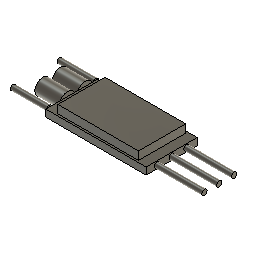
Battle bot V3,6 (Autodesk Fusion 360 archive; units mm, degrees)
design "40a esc brushless"
Autodesk Fusion 360 part; units mm, degrees
sketch "Sketch1" plane through (0, 0, 0) normal (0, 0, 1) x (1, 0, 0)
  line L0 (0, 0) -> (52.74, 0)
  line L1 (52.74, 0) -> (52.74, 26.87)
  line L2 (52.74, 26.87) -> (0, 26.87)
  line L3 (0, 26.87) -> (0, 0)
  dimension "d1" = 52.74
  dimension "d2" = 26.87
  constraint horizontal L0
  constraint vertical L1
  constraint horizontal L2
  constraint vertical L3
  constraint coincident L0.start L3.end
  measures "d1" distance of L0.start L0.end
  measures "d2" distance of L0 L2
extrude "Extrude1" add sketch "Sketch1" along normal blind 3.7
sketch "Sketch2" plane through (0, 0, 0) normal (-1, 0, 0) x (0, -1, 0)
  line L0 (-26.87, 0) -> (0, 0)
  line L1 (0, 0) -> (0, 3.7)
  line L2 (0, 3.7) -> (-26.87, 3.7)
  line L3 (-26.87, 3.7) -> (-26.87, 0)
  circle A0 centre (-20.65, 1.85) radius 4.12
  line L4 (-20.65, 1.85) -> (-11.35, 1.85) construction
  circle A1 centre (-11.35, 1.85) radius 4.12
  circle A2 centre (-26.2658, 3.1834) radius 1.4
  circle A3 centre (-1.7767, 3.1834) radius 1.4
  dimension "d5" = 8.24
  dimension "d6" = 6.22
  dimension "d7" = 9.3
  dimension "d8" = 8.24
  dimension "d9" = 2.8
  dimension "d10" = 2.8
  constraint coincident A0.centre L4.start
  constraint perpendicular L1 L4
  constraint coincident L4.end A1.centre
  measures "d5" diameter of A0
  measures "d6" distance of L3 A0.centre
  measures "d7" distance of A0.centre L4.end
  measures "d8" diameter of A1
  measures "d9" diameter of A2
  measures "d10" diameter of A3
extrude "Extrude2" add sketch "Sketch2" along normal blind 13 contours L0 L2 A0 | L0 A0 | L2 L3 A2 | L2 L3 A2 | L2 A0 | L0 L2 A1 | L0 A1 | L2 A1 | L2 A3 | L2 A3
extrude "Extrude3" add 2 faces at (-13, 26.6777, 2.866) (-13, 1.2269, 3.5008) along direction (-1, 0, 0) blind 6
sketch "Sketch3" plane through (0, 0, 3.7) normal (0, 0, 1) x (-1, 0, 0)
  line L0 (0, -26.87) -> (0, -24.9646)
  line L1 (0, -24.9646) -> (0, -24.3313)
  line L2 (0, -24.3313) -> (0, -16.9687)
  line L3 (0, -16.9687) -> (0, -15.0313)
  line L4 (0, -15.0313) -> (0, -7.6687)
  line L5 (0, -7.6687) -> (0, -3.0779)
  line L6 (0, -3.0779) -> (0, -0.4755)
  line L7 (0, -0.4755) -> (0, 0)
  line L8 (0, 0) -> (-52.74, 0)
  line L9 (-52.74, 0) -> (-52.74, -26.87)
  line L10 (-52.74, -26.87) -> (0, -26.87)
  line L11 (-47.74, -1) -> (-5.34, -1)
  line L12 (-5.34, -1) -> (-5.34, -25.76)
  line L13 (-5.34, -25.76) -> (-47.74, -25.76)
  line L14 (-47.74, -25.76) -> (-47.74, -1)
  dimension "d15" = 24.76
  dimension "d16" = 1
  dimension "d17" = 42.4
  dimension "d18" = 5
  constraint horizontal L11
  constraint vertical L12
  constraint horizontal L13
  constraint vertical L14
  measures "d15" distance of L11 L13
  measures "d16" distance of L8 L11
  measures "d17" distance of L12 L14
  measures "d18" distance of L9 L14
extrude "Extrude4" add sketch "Sketch3" along normal blind 4.3 contours L11 L12 L13 L14
sketch "Sketch4" plane through (52.74, 0, 0) normal (1, 0, 0) x (0, 1, 0)
  line L0 (0, 0) -> (26.87, 0)
  line L1 (26.87, 0) -> (26.87, 3.7)
  line L2 (26.87, 3.7) -> (0, 3.7)
  line L3 (0, 3.7) -> (0, 0)
  circle A0 centre (13.435, 1.85) radius 1.4
  line L4 (14.835, 1.85) -> (19.835, 1.85) construction
  circle A1 centre (21.235, 1.85) radius 1.4
  line L5 (13.435, 1.85) -> (13.435, 3.7) construction
  circle A2 centre (5.635, 1.85) radius 1.4
  dimension "d21" = 2.8
  dimension "d22" = 5
  dimension "d23" = 2.8
  constraint coincident A0 L4.start
  constraint parallel L2 L4
  constraint coincident L4.end A1
  constraint coincident A0.centre L5.start
  constraint midpoint L2 L5.end
  constraint perpendicular L2 L5
  constraint symmetric A1 L5 A2
  measures "d21" diameter of A0
  measures "d22" distance of L4.start L4.end
  measures "d23" diameter of A1
extrude "Extrude5" add sketch "Sketch4" along normal blind 25 contours A0 | A1 | A2

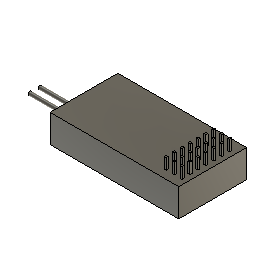
design "Reciever"
Autodesk Fusion 360 part; units mm, degrees
sketch "Sketch1" plane through (0, 0, 0) normal (0, 0, 1) x (1, 0, 0)
  line L0 (0, 0) -> (41.17, 0)
  line L1 (41.17, 0) -> (41.17, 21.69)
  line L2 (41.17, 21.69) -> (0, 21.69)
  line L3 (0, 21.69) -> (0, 0)
  dimension "d1" = 41.17
  dimension "d2" = 21.69
  constraint horizontal L0
  constraint vertical L1
  constraint horizontal L2
  constraint vertical L3
  constraint coincident L0.start L3.end
  measures "d1" distance of L0.start L0.end
  measures "d2" distance of L0.start L2.end
extrude "Extrude1" add sketch "Sketch1" along normal blind 8.92
sketch "Sketch2" plane through (0, 0, 8.92) normal (0, 0, 1) x (-1, 0, 0)
  line L0 (0, -21.69) -> (0, 0)
  line L1 (0, 0) -> (-41.17, 0)
  line L2 (-41.17, 0) -> (-41.17, -21.69)
  line L3 (-41.17, -21.69) -> (0, -21.69)
  line L4 (-33.97, -18.44) -> (-39.67, -18.44)
  line L5 (-39.67, -18.44) -> (-39.67, -2.54)
  line L6 (-39.67, -2.54) -> (-33.97, -2.54)
  line L7 (-33.97, -2.54) -> (-33.97, -18.44)
  line L8 (-39.67, -18.44) -> (-39.02, -18.44)
  line L9 (-39.02, -18.44) -> (-39.02, -17.79)
  line L10 (-39.02, -17.79) -> (-39.67, -17.79)
  line L11 (-39.67, -17.79) -> (-39.67, -18.44)
  line L12 (-37.145, -18.44) -> (-36.495, -18.44)
  line L13 (-36.495, -18.44) -> (-36.495, -17.79)
  line L14 (-37.145, -17.79) -> (-37.145, -18.44)
  line L15 (-36.495, -17.79) -> (-37.145, -17.79)
  line L16 (-34.62, -18.44) -> (-33.97, -18.44)
  line L17 (-33.97, -18.44) -> (-33.97, -17.79)
  line L18 (-34.62, -17.79) -> (-34.62, -18.44)
  line L19 (-33.97, -17.79) -> (-34.62, -17.79)
  line L20 (-39.67, -15.8983) -> (-39.02, -15.8983)
  line L21 (-39.02, -15.8983) -> (-39.02, -15.2483)
  line L22 (-39.67, -15.2483) -> (-39.67, -15.8983)
  line L23 (-39.02, -15.2483) -> (-39.67, -15.2483)
  line L24 (-37.145, -15.8983) -> (-36.495, -15.8983)
  line L25 (-36.495, -15.8983) -> (-36.495, -15.2483)
  line L26 (-37.145, -15.2483) -> (-37.145, -15.8983)
  line L27 (-36.495, -15.2483) -> (-37.145, -15.2483)
  line L28 (-34.62, -15.8983) -> (-33.97, -15.8983)
  line L29 (-33.97, -15.8983) -> (-33.97, -15.2483)
  line L30 (-34.62, -15.2483) -> (-34.62, -15.8983)
  line L31 (-33.97, -15.2483) -> (-34.62, -15.2483)
  line L32 (-39.67, -13.3567) -> (-39.02, -13.3567)
  line L33 (-39.02, -13.3567) -> (-39.02, -12.7067)
  line L34 (-39.67, -12.7067) -> (-39.67, -13.3567)
  line L35 (-39.02, -12.7067) -> (-39.67, -12.7067)
  line L36 (-37.145, -13.3567) -> (-36.495, -13.3567)
  line L37 (-36.495, -13.3567) -> (-36.495, -12.7067)
  line L38 (-37.145, -12.7067) -> (-37.145, -13.3567)
  line L39 (-36.495, -12.7067) -> (-37.145, -12.7067)
  line L40 (-34.62, -13.3567) -> (-33.97, -13.3567)
  line L41 (-33.97, -13.3567) -> (-33.97, -12.7067)
  line L42 (-34.62, -12.7067) -> (-34.62, -13.3567)
  line L43 (-33.97, -12.7067) -> (-34.62, -12.7067)
  line L44 (-39.67, -10.815) -> (-39.02, -10.815)
  line L45 (-39.02, -10.815) -> (-39.02, -10.165)
  line L46 (-39.67, -10.165) -> (-39.67, -10.815)
  line L47 (-39.02, -10.165) -> (-39.67, -10.165)
  line L48 (-37.145, -10.815) -> (-36.495, -10.815)
  line L49 (-36.495, -10.815) -> (-36.495, -10.165)
  line L50 (-37.145, -10.165) -> (-37.145, -10.815)
  line L51 (-36.495, -10.165) -> (-37.145, -10.165)
  line L52 (-34.62, -10.815) -> (-33.97, -10.815)
  line L53 (-33.97, -10.815) -> (-33.97, -10.165)
  line L54 (-34.62, -10.165) -> (-34.62, -10.815)
  line L55 (-33.97, -10.165) -> (-34.62, -10.165)
  line L56 (-39.67, -8.2733) -> (-39.02, -8.2733)
  line L57 (-39.02, -8.2733) -> (-39.02, -7.6233)
  line L58 (-39.67, -7.6233) -> (-39.67, -8.2733)
  line L59 (-39.02, -7.6233) -> (-39.67, -7.6233)
  line L60 (-37.145, -8.2733) -> (-36.495, -8.2733)
  line L61 (-36.495, -8.2733) -> (-36.495, -7.6233)
  line L62 (-37.145, -7.6233) -> (-37.145, -8.2733)
  line L63 (-36.495, -7.6233) -> (-37.145, -7.6233)
  line L64 (-34.62, -8.2733) -> (-33.97, -8.2733)
  line L65 (-33.97, -8.2733) -> (-33.97, -7.6233)
  line L66 (-34.62, -7.6233) -> (-34.62, -8.2733)
  line L67 (-33.97, -7.6233) -> (-34.62, -7.6233)
  line L68 (-39.67, -5.7317) -> (-39.02, -5.7317)
  line L69 (-39.02, -5.7317) -> (-39.02, -5.0817)
  line L70 (-39.67, -5.0817) -> (-39.67, -5.7317)
  line L71 (-39.02, -5.0817) -> (-39.67, -5.0817)
  line L72 (-37.145, -5.7317) -> (-36.495, -5.7317)
  line L73 (-36.495, -5.7317) -> (-36.495, -5.0817)
  line L74 (-37.145, -5.0817) -> (-37.145, -5.7317)
  line L75 (-36.495, -5.0817) -> (-37.145, -5.0817)
  line L76 (-34.62, -5.7317) -> (-33.97, -5.7317)
  line L77 (-33.97, -5.7317) -> (-33.97, -5.0817)
  line L78 (-34.62, -5.0817) -> (-34.62, -5.7317)
  line L79 (-33.97, -5.0817) -> (-34.62, -5.0817)
  line L80 (-39.67, -3.19) -> (-39.02, -3.19)
  line L81 (-39.02, -3.19) -> (-39.02, -2.54)
  line L82 (-39.67, -2.54) -> (-39.67, -3.19)
  line L83 (-39.02, -2.54) -> (-39.67, -2.54)
  line L84 (-37.145, -3.19) -> (-36.495, -3.19)
  line L85 (-36.495, -3.19) -> (-36.495, -2.54)
  line L86 (-37.145, -2.54) -> (-37.145, -3.19)
  line L87 (-36.495, -2.54) -> (-37.145, -2.54)
  line L88 (-34.62, -3.19) -> (-33.97, -3.19)
  line L89 (-33.97, -3.19) -> (-33.97, -2.54)
  line L90 (-34.62, -2.54) -> (-34.62, -3.19)
  line L91 (-33.97, -2.54) -> (-34.62, -2.54)
  dimension "d5" = 5.7
  dimension "d6" = 15.9
  dimension "d7" = 1.5
  dimension "d8" = 3.25
  dimension "d9" = 0.65
  dimension "d10" = 0.65
  dimension "d13" = 5.05
  dimension "d14" = 15.25
  constraint horizontal L4
  constraint vertical L5
  constraint horizontal L6
  constraint vertical L7
  constraint horizontal L8
  constraint vertical L9
  constraint horizontal L10
  constraint vertical L11
  measures "d5" distance of L4.start L4.end
  measures "d6" distance of L4.start L6.end
  measures "d7" distance of L2 L5
  measures "d8" distance of L3 L4
  measures "d9" distance of L4.end L8.end
  measures "d10" distance of L4.end L10.end
extrude "Extrude2" add sketch "Sketch2" along normal blind 3.5 contours L4 L7 L16 L17 L18 L19 | L4 L12 L13 L14 L15 | L7 L28 L29 L30 L31 | L4 L5 L8 L9 L10 L11 | L7 L40 L41 L42 L43 | L7 L52 L53 L54 L55 | L5 L20 L21 L22 L23 | L7 L64 L65 L66 L67 | L5 L32 L33 L34 L35 | L7 L76 L77 L78 L79 | L5 L44 L45 L46 L47 | L6 L7 L88 L89 L90 L91 | L5 L56 L57 L58 L59 | L5 L68 L69 L70 L71 | L6 L84 L85 L86 L87 | L5 L6 L80 L81 L82 L83 | L24 L25 L26 L27 | L36 L37 L38 L39 | L48 L49 L50 L51 | L60 L61 L62 L63 | L72 L73 L74 L75
sketch "Sketch3" plane through (0, 0, 0) normal (-1, 0, 0) x (0, -1, 0)
  line L0 (-21.69, 0) -> (0, 0)
  line L1 (0, 0) -> (0, 8.92)
  line L2 (0, 8.92) -> (-21.69, 8.92)
  line L3 (-21.69, 8.92) -> (-21.69, 0)
  circle A0 centre (-9.85, 4.4059) radius 0.6
  circle A1 centre (-6.57, 4.4059) radius 0.6
  line L4 (-5.97, 4.4059) -> (-10.45, 4.4059) construction
  dimension "d17" = 1.2
  dimension "d18" = 11.84
  dimension "d19" = 1.2
  dimension "d20" = 4.48
  constraint coincident A1 L4.start
  constraint coincident A0 L4.end
  constraint horizontal L4
  measures "d17" diameter of A0
  measures "d18" distance of L3 A0.centre
  measures "d19" diameter of A1
  measures "d20" distance of L4.start L4.end
extrude "Extrude3" add sketch "Sketch3" along normal blind 13 contours A0 | A1

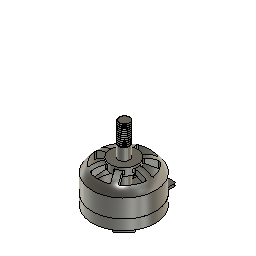
design "Weapon motor"
Autodesk Fusion 360 part; units mm, degrees
sketch "Sketch1" plane through (0, 0, 0) normal (0, 0, 1) x (1, 0, 0)
  circle A0 centre (0, 0) radius 2.5
  dimension "d1" = 5
  constraint coincident A0.centre origin
  measures "d1" diameter of A0
extrude "Extrude1" add sketch "Sketch1" along normal blind 33.45 makes body 1
ref_plane "WorkPlane1" through (0, 0, 19.34) normal (0, 0, 1) x (1, 0, 0)
sketch "Sketch2" plane through (0, 0, 19.34) normal (0, 0, 1) x (1, 0, 0)
  circle A0 centre (0, 0) radius 5.935
  dimension "d5" = 11.87
  constraint coincident A0.centre origin
  measures "d5" diameter of A0
extrude "Extrude2" add sketch "Sketch2" against normal blind 0.98 bodies 1
sketch "Sketch3" plane through (0, 0, 18.36) normal (0, 0, -1) x (1, 0, 0)
  circle A0 centre (0, 0) radius 5.935
  circle A1 centre (0, 0) radius 2.5
  circle A2 centre (0, 0) radius 13.905
  dimension "d8" = 27.81
  constraint concentric A0 A2
  measures "d8" diameter of A2
ref_plane "WorkPlane2" through (0, 0, 45.735) normal (0, 1, 0) x (0, 0, 1)
sketch "Sketch4" plane through (0, 0, 45.735) normal (0, 1, 0) x (1, 0, 0)
  line L0 (-2.5, 26.395) -> (2.5, 26.395)
  line L1 (-2.5, 12.285) -> (2.5, 12.285)
  line L2 (5.935, 27.375) -> (-5.935, 27.375)
  line L3 (-5.935, 26.395) -> (5.935, 26.395)
  line L4 (-2.5, 45.735) -> (2.5, 45.735)
  line L5 (2.5, 27.375) -> (-2.5, 27.375)
  line L6 (2.5, 27.375) -> (2.5, 32.315) construction
  line L7 (0, 27.375) -> (13.9, 27.375) construction
  line L8 (-2.5, 26.395) -> (-2.5, 45.645) construction
  line L9 (-2.5, 45.735) -> (-2.5, 43.865) construction
  line L10 (13.9, 32.315) -> (13.9, 40.315)
  arc A0 (5.935, 27.375) -> (13.9, 32.315) centre (5.935, 36.2662) ccw
  line L11 (11.4, 32.315) -> (11.4, 40.315)
  line L12 (5.935, 28.905) -> (11.4, 32.315)
  line L13 (5.935, 27.375) -> (5.935, 29.6599)
  line L14 (5.935, 29.6599) -> (2.7365, 29.6599)
  line L15 (2.7365, 29.6599) -> (2.7365, 27.375)
  line L16 (13.9, 40.315) -> (11.4, 40.315)
  dimension "d12" = 4.94
  dimension "d13" = 13.9
  dimension "d14" = 19.25
  dimension "d15" = 1.87
  dimension "d16" = -2.5
  dimension "d29" = 8
  dimension "d30" = 4.94
  constraint coincident L5.start L6.start
  constraint perpendicular L5 L6
  constraint midpoint L2 L7.start
  constraint parallel L2 L7
  constraint coincident L0.start L8.start
  constraint perpendicular L5 L8
  constraint coincident L4.start L9.start
  constraint perpendicular L4 L9
  constraint perpendicular L7 L10
  constraint tangent L7 A0
  constraint coincident L2.start A0.start
  constraint perpendicular L7 L13
  constraint perpendicular L6 L14
  constraint coincident L2 L15.end
  constraint vertical L15
  measures "d12" distance of L5.start L6.end
  measures "d13" distance of L7.start L7.end
  measures "d14" distance of L0.start L8.end
  measures "d15" distance of L4.start L9.end
  measures "d29" distance of L10.end L10.start
  measures "d30" vertical distance of L2.start L10.start
revolve "Revolve1" add sketch "Sketch4" angle 360 about axis through (0, 0, 31.625) along (0, 0, 1) bodies 1
sketch "Sketch6" plane through (0, 0, 19.34) normal (0, 0, 1) x (-1, 0, 0)
  circle A0 centre (0, 0) radius 5.935
  circle A1 centre (0, 0) radius 2.5
  circle A2 centre (0, 0) radius 11.4
  circle A3 centre (0, 0) radius 13.9
  line L0 (5.935, 0) -> (11.4, 0) construction
  line L1 (10.8574, -1.25) -> (6.2331, -1.25)
  arc A4 (11.2693, -1.7216) -> (10.8574, -1.25) centre (10.8574, -1.6656) ccw
  arc A5 (6.2699, -1.25) -> (5.6965, -1.6656) centre (6.2515, -1.8279) ccw
  line L2 (10.8574, 1.25) -> (6.2331, 1.25)
  arc A6 (10.8574, 1.25) -> (11.2693, 1.7216) centre (10.8574, 1.6656) ccw
  arc A7 (5.6965, 1.6656) -> (6.2699, 1.25) centre (6.2515, 1.8279) ccw
  line L3 (6.5112, 8.7778) -> (4.1991, 4.773)
  arc A8 (4.2175, 4.8049) -> (4.2907, 4.1005) centre (4.7088, 4.5) ccw
  arc A9 (7.1256, 8.8987) -> (6.5112, 8.7778) centre (6.8712, 8.57) ccw
  arc A10 (1.4057, 5.7661) -> (2.0524, 6.0549) centre (1.5427, 6.3279) ccw
  line L4 (2.9675, 5.1399) -> (5.7, 9.8727) construction
  line L5 (4.3462, 10.0278) -> (2.034, 6.023)
  arc A11 (4.3462, 10.0278) -> (4.1437, 10.6203) centre (3.9862, 10.2356) ccw
  line L6 (-4.3462, 10.0278) -> (-2.034, 6.023)
  arc A12 (-2.0524, 6.0549) -> (-1.4057, 5.7661) centre (-1.5427, 6.3279) ccw
  arc A13 (-4.1437, 10.6203) -> (-4.3462, 10.0278) centre (-3.9862, 10.2356) ccw
  arc A14 (-4.2907, 4.1005) -> (-4.2175, 4.8049) centre (-4.7088, 4.5) ccw
  line L7 (-2.9675, 5.1399) -> (-5.7, 9.8727) construction
  line L8 (-6.5112, 8.7778) -> (-4.1991, 4.773)
  arc A15 (-6.5112, 8.7778) -> (-7.1256, 8.8987) centre (-6.8712, 8.57) ccw
  line L9 (-10.8574, 1.25) -> (-6.2331, 1.25)
  arc A16 (-6.2699, 1.25) -> (-5.6965, 1.6656) centre (-6.2515, 1.8279) ccw
  arc A17 (-11.2693, 1.7216) -> (-10.8574, 1.25) centre (-10.8574, 1.6656) ccw
  arc A18 (-5.6965, -1.6656) -> (-6.2699, -1.25) centre (-6.2515, -1.8279) ccw
  line L10 (-5.935, 0) -> (-11.4, 0) construction
  line L11 (-10.8574, -1.25) -> (-6.2331, -1.25)
  arc A19 (-10.8574, -1.25) -> (-11.2693, -1.7216) centre (-10.8574, -1.6656) ccw
  line L12 (-6.5112, -8.7778) -> (-4.1991, -4.773)
  arc A20 (-4.2175, -4.8049) -> (-4.2907, -4.1005) centre (-4.7088, -4.5) ccw
  arc A21 (-7.1256, -8.8987) -> (-6.5112, -8.7778) centre (-6.8712, -8.57) ccw
  arc A22 (-1.4057, -5.7661) -> (-2.0524, -6.0549) centre (-1.5427, -6.3279) ccw
  line L13 (-2.9675, -5.1399) -> (-5.7, -9.8727) construction
  line L14 (-4.3462, -10.0278) -> (-2.034, -6.023)
  arc A23 (-4.3462, -10.0278) -> (-4.1437, -10.6203) centre (-3.9862, -10.2356) ccw
  line L15 (4.3462, -10.0278) -> (2.034, -6.023)
  arc A24 (2.0524, -6.0549) -> (1.4057, -5.7661) centre (1.5427, -6.3279) ccw
  arc A25 (4.1437, -10.6203) -> (4.3462, -10.0278) centre (3.9862, -10.2356) ccw
  arc A26 (4.2907, -4.1005) -> (4.2175, -4.8049) centre (4.7088, -4.5) ccw
  line L16 (2.9675, -5.1399) -> (5.7, -9.8727) construction
  line L17 (6.5112, -8.7778) -> (4.1991, -4.773)
  arc A27 (6.5112, -8.7778) -> (7.1256, -8.8987) centre (6.8712, -8.57) ccw
  circle A28 centre (0, 0) radius 5.935
  circle A29 centre (0, 0) radius 2.5
  dimension "d24" = 1.25
  dimension "d26" = 360
  constraint coincident A0 L0.start
  constraint coincident A2 L0.end
  constraint horizontal L0
  constraint parallel L0 L1
  constraint tangent L1 A4
  constraint coincident A2 A4.start
  constraint tangent A0 A5
  constraint coincident A0 A5.end
  constraint coincident L1 A5.start
  constraint coincident A5 L1.end
  constraint symmetric L0 L1.start L2.start
  constraint symmetric L0 A4.start A6.end
  constraint symmetric L0 A4 A6
  constraint symmetric L0 A5.start A7.end
  constraint symmetric L0 A5.end A7.start
  constraint symmetric L0 A5 A7
  constraint symmetric L0 L1.end L2.end
  measures "d24" distance of L0 L1
extrude "Extrude4" cut sketch "Sketch6" against normal blind 7 contours A0 A2 L2 A6 A7 L3 A8 A9 A28 | A0 A2 L1 A4 A5 A26 L17 A27 A28 | A0 A2 A10 L5 A11 L6 A12 A13 A28 | A0 A2 A22 L14 A23 L15 A24 A25 A28 | A0 A2 A14 L8 A15 L9 A16 A17 A28 | A0 A2 A18 L11 A19 L12 A20 A21 A28 bodies 1
extrude "Extrude5" add 1 faces at (9.4162, -9.0112, 5.42) along direction (0, 0, -1) blind 4.5 separate body on bodies 1 makes body 2
sketch "Sketch8" plane through (0, 0, 0.92) normal (0, 0, -1) x (1, 0, 0)
  circle A0 centre (0, 0) radius 11.4
  circle A1 centre (0, 0) radius 13.9
  circle A2 centre (0, 0) radius 5.25
  circle A3 centre (0, 0) radius 6.5
  circle A4 centre (0, 0) radius 12.5
  line L0 (0, 0) -> (8.8388, 8.8388) construction
  line L1 (0, 0) -> (12.5, 0) construction
  line L2 (6.3479, 1.3981) -> (10.9602, 6.0104)
  line L3 (1.3981, 6.3479) -> (6.0104, 10.9602)
  line L4 (-6.3479, 1.3981) -> (-10.9602, 6.0104)
  line L5 (-1.3981, 6.3479) -> (-6.0104, 10.9602)
  line L6 (0, 0) -> (-8.8388, 8.8388) construction
  line L7 (-1.3981, -6.3479) -> (-6.0104, -10.9602)
  line L8 (-6.3479, -1.3981) -> (-10.9602, -6.0104)
  line L9 (0, 0) -> (-8.8388, -8.8388) construction
  line L10 (6.3479, -1.3981) -> (10.9602, -6.0104)
  line L11 (1.3981, -6.3479) -> (6.0104, -10.9602)
  line L12 (0, 0) -> (8.8388, -8.8388) construction
  line L13 (0, 0) -> (-4.8684, 4.8684) construction
  circle A5 centre (-5.7523, 5.7523) radius 1.25
  circle A6 centre (5.7523, -5.7523) radius 1.25
  line L14 (0, 0) -> (5.9008, 5.9008) construction
  circle A7 centre (6.7847, 6.7847) radius 1.25
  circle A8 centre (-6.7847, -6.7847) radius 1.25
  line L15 (0, 0) -> (10.44, 0) construction
  line L16 (8.345, 2.095) -> (7.0447, 2.095)
  line L17 (8.345, -2.095) -> (7.0447, -2.095)
  arc A9 (8.345, -2.095) -> (8.345, 2.095) centre (8.345, 0) ccw
  line L18 (0, -2.5) -> (0, -20)
  line L19 (-8.345, 2.095) -> (-7.0447, 2.095)
  arc A10 (-8.345, 2.095) -> (-8.345, -2.095) centre (-8.345, 0) ccw
  line L20 (-8.345, -2.095) -> (-7.0447, -2.095)
  circle A11 centre (-5.7523, 5.7523) radius 1.3
  circle A12 centre (6.7847, 6.7847) radius 1.3
  circle A13 centre (5.7523, -5.7523) radius 1.3
  circle A14 centre (-6.7847, -6.7847) radius 1.3
  dimension "d33" = 10.5
  dimension "d34" = 13
  dimension "d35" = 25
  dimension "d36" = 45
  dimension "d37" = 3.5
  dimension "d39" = 360
  dimension "d40" = 6.885
  dimension "d41" = 2.5
  dimension "d42" = 8.345
  dimension "d43" = 2.5
  dimension "d44" = 10.44
  dimension "d62" = 2.6
  dimension "d63" = 2.6
  dimension "d64" = 2.6
  dimension "d65" = 2.6
  constraint coincident A0.centre A1.centre
  constraint concentric A2 A3
  constraint concentric A2 A4
  constraint horizontal L1
  constraint coincident A4 L0.end
  constraint parallel L0 L2
  constraint coincident A3 L2.start
  constraint coincident A4 L2.end
  constraint symmetric L0 L2.start L3.start
  constraint symmetric L0 L2.end L3.end
  constraint parallel L6 L13
  constraint coincident L13.end A5
  constraint symmetric L0 A5 A6
  constraint perpendicular L13 L14
  constraint coincident L14.end A7
  constraint symmetric L12 A7 A8
  constraint parallel L1 L15
  constraint coincident L15.end A9
  constraint coincident L2 L16.end
  constraint tangent L16 A9
  constraint parallel L15 L16
  constraint coincident L10 L17.end
  constraint tangent L17 A9
  constraint parallel L15 L17
  constraint symmetric L16.start L18 L19.start
  constraint symmetric L16.end L18 L19.end
  constraint symmetric L17.start L18 A10.end
  constraint symmetric L17.end L18 L20.end
  constraint symmetric A9 L18 A10
  constraint concentric A5 A11
  constraint concentric A7 A12
  constraint concentric A6 A13
  constraint concentric A8 A14
  measures "d33" diameter of A2
  measures "d34" diameter of A3
  measures "d35" diameter of A4
  measures "d36" angle of L0 L1
  measures "d37" distance of L0 L2
  measures "d40" distance of A0.centre L13.end
  measures "d41" diameter of A5
  measures "d42" distance of A0.centre L14.end
  measures "d43" diameter of A7
  measures "d44" distance of A0.centre L15.end
  measures "d62" diameter of A11
  measures "d63" diameter of A12
  measures "d64" diameter of A13
  measures "d65" diameter of A14
extrude "Extrude6" add sketch "Sketch8" along normal blind 1.85 contours A0 A3 L2 L3 | A0 A4 L2 L3 | A0 A4 L10 L11 | A0 A3 L10 L11 | A3 L2 L10 L16 L17 A9 | A0 A3 L4 L5 | A0 A4 L4 L5 | A3 | A0 A4 L7 L8 | A0 A3 L7 L8 | A3 L4 L8 L19 A10 L20 bodies 2
sketch "Sketch9" plane through (0, 0, 0.92) normal (0, 0, -1) x (1, 0, 0)
  line L0 (-6.0104, 10.9602) -> (-5.1968, 10.1466)
  arc A0 (5.1968, 10.1466) -> (-5.1968, 10.1466) centre (0, 0) ccw
  line L1 (5.1968, 10.1466) -> (6.0104, 10.9602)
  arc A1 (10.9602, 6.0104) -> (6.0104, 10.9602) centre (0, 0) ccw
  line L2 (10.9602, 6.0104) -> (10.1466, 5.1968)
  arc A2 (10.1466, -5.1968) -> (10.1466, 5.1968) centre (0, 0) ccw
  line L3 (10.1466, -5.1968) -> (10.9602, -6.0104)
  arc A3 (6.0104, -10.9602) -> (10.9602, -6.0104) centre (0, 0) ccw
  line L4 (6.0104, -10.9602) -> (5.1968, -10.1466)
  arc A4 (-5.1968, -10.1466) -> (5.1968, -10.1466) centre (0, 0) ccw
  line L5 (-5.1968, -10.1466) -> (-6.0104, -10.9602)
  arc A5 (-10.9602, -6.0104) -> (-6.0104, -10.9602) centre (0, 0) ccw
  line L6 (-10.9602, -6.0104) -> (-10.1466, -5.1968)
  arc A6 (-10.1466, 5.1968) -> (-10.1466, -5.1968) centre (0, 0) ccw
  line L7 (-10.1466, 5.1968) -> (-10.9602, 6.0104)
  arc A7 (-6.0104, 10.9602) -> (-10.9602, 6.0104) centre (0, 0) ccw
  circle A8 centre (0, 0) radius 13.9
  circle A9 centre (0, 0) radius 5.25 construction
  arc A10 (-8.345, 2.095) -> (-8.345, -2.095) centre (-8.345, 0) ccw construction
  line L8 (-8.345, -2.095) -> (-7.0447, -2.095) construction
  line L9 (-7.0447, -2.095) -> (-10.9602, -6.0104) construction
  arc A11 (-10.9602, -6.0104) -> (-6.0104, -10.9602) centre (0, 0) ccw construction
  line L10 (-6.0104, -10.9602) -> (-1.3981, -6.3479) construction
  arc A12 (-1.3981, -6.3479) -> (1.3981, -6.3479) centre (0, 0) ccw construction
  line L11 (1.3981, -6.3479) -> (6.0104, -10.9602) construction
  arc A13 (6.0104, -10.9602) -> (10.9602, -6.0104) centre (0, 0) ccw construction
  line L12 (10.9602, -6.0104) -> (7.0447, -2.095) construction
  line L13 (7.0447, -2.095) -> (8.345, -2.095) construction
  arc A14 (8.345, -2.095) -> (8.345, 2.095) centre (8.345, 0) ccw construction
  line L14 (8.345, 2.095) -> (7.0447, 2.095) construction
  line L15 (7.0447, 2.095) -> (10.9602, 6.0104) construction
  arc A15 (10.9602, 6.0104) -> (6.0104, 10.9602) centre (0, 0) ccw construction
  line L16 (6.0104, 10.9602) -> (1.3981, 6.3479) construction
  arc A16 (1.3981, 6.3479) -> (-1.3981, 6.3479) centre (0, 0) ccw construction
  line L17 (-1.3981, 6.3479) -> (-6.0104, 10.9602) construction
  arc A17 (-6.0104, 10.9602) -> (-10.9602, 6.0104) centre (0, 0) ccw construction
  line L18 (-10.9602, 6.0104) -> (-7.0447, 2.095) construction
  line L19 (-7.0447, 2.095) -> (-8.345, 2.095) construction
  line L20 (0, -5.25) -> (0, -13.9) construction
  line L21 (0, -17.55) -> (5.555, -17.55)
  line L22 (5.555, -17.55) -> (5.555, -5.8964)
  line L23 (5.555, -5.8964) -> (0, -5.8964)
  line L24 (-5.555, -17.55) -> (-5.555, -5.8964)
  line L25 (-5.555, -5.8964) -> (0, -5.8964)
  line L26 (0, -17.55) -> (-5.555, -17.55)
  line L27 (0, -5.8964) -> (0, -6.5)
  circle A18 centre (5.7523, -5.7523) radius 1.3
  circle A19 centre (6.7847, 6.7847) radius 1.3
  circle A20 centre (-6.7847, -6.7847) radius 1.3
  circle A21 centre (-5.7523, 5.7523) radius 1.3
  dimension "d53" = 12.3
  dimension "d54" = 5.555
  constraint coincident A9 L20.start
  constraint vertical L20
  constraint horizontal L21
  constraint vertical L22
  constraint horizontal L23
  constraint vertical L27
  constraint symmetric L21.start L26.start L27
  constraint symmetric L21.end L24.start L27
  constraint symmetric L22.end L24.end L27
  constraint coincident A8 L20.end
  constraint coincident A12 L27.end
  measures "d53" distance of L20.start L21.start
  measures "d54" distance of L21.start L21.end
extrude "Extrude7" cut sketch "Sketch9" against normal blind 3.48 contours L4 A4 L5 L22 L23 L24 L25 A18 A20 | L4 A4 L5 A8 L22 L24 | A8 L21 L22 L24 L26 | L24 A20 | L22 L23 A18 picked at (-5.542, -6.69) picked at (4.9828, -6.3022) bodies 2
extrude "Extrude8" add sketch "Sketch9" against normal blind 1.1 from surface at -1.45 contours L4 A4 L5 L22 L23 L24 L25 A18 A20 | L4 A4 L5 A8 L22 L24 | A8 L21 L22 L24 L26 | L24 A20 | L22 L23 A18 picked at (-5.542, -6.69) picked at (4.9828, -6.3022) bodies 2
fillet "Fillet1" radius 0.75 2 edges at (-5.555, 17.55, 2.92) (5.555, 17.55, 2.92) on bodies 2
copy_body "Body->Comp1" bodies 1 removing the originals makes body 3 in component "Component"
copy_body "Body->Comp2" bodies 2 removing the originals makes body 4 in component "Component'"
thread "Thread1" "ISO Metric profile 5.0 M5x0.8 6g" major diameter 4.901 minor diameter 3.9895 pitch 0.8 angle 60 modelled left hand crest width 0.1157 on face at (2.4676, 0.401, 24.0433) from (0, 0, 24.55) to (0, 0, 33.45) crest through (2.4505, 0, 19.14) on bodies 3 in component "Component"
component "Component" placed x (1, 0, 0) y (0, 1, 0) z (0, 0, 1) at (0, 0, 0)
component "Component'" placed x (1, 0, 0) y (0, 1, 0) z (0, 0, 1) at (0, 0, 0)
equation "d12 = 6.09 mm - 1.15 mm"
equation "d13 = ( 27.8 / 2 ) * 1 mm"
equation "d24 = ( 2.5 / 2 ) * 1 mm"
equation "d40 = ( 13.77 / 2 ) * 1 mm"
equation "d42 = ( 16.69 / 2 ) * 1 mm"
equation "d44 = ( 20.88 / 2 ) * 1 mm"
equation "d54 = ( 11.11 / 2 ) * 1 mm"

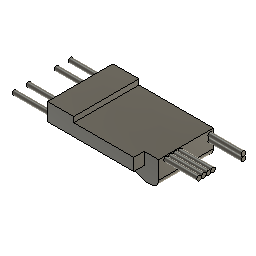
design "dual motor esc"
Autodesk Fusion 360 part; units mm, degrees
sketch "Sketch1" plane through (0, 0, 0) normal (0, 0, 1) x (1, 0, 0)
  line L0 (0, 0) -> (33.8, 0)
  line L1 (33.8, 0) -> (33.8, 25.6)
  line L2 (33.8, 25.6) -> (0, 25.6)
  line L3 (0, 25.6) -> (0, 0)
  line L4 (0, 21.3068) -> (39.45, 21.3068) construction
  line L5 (39.45, 25.6) -> (33.8, 25.6)
  line L6 (33.8, 25.6) -> (33.8, 4.1)
  line L7 (33.8, 4.1) -> (39.45, 4.1)
  line L8 (39.45, 4.1) -> (39.45, 25.6)
  line L9 (0, 25.6) -> (10.24, 25.6)
  line L10 (10.24, 25.6) -> (10.24, 0)
  line L11 (10.24, 0) -> (0, 0)
  line L12 (0, 0) -> (0, 25.6)
  dimension "d1" = 33.8
  dimension "d2" = 25.6
  dimension "d3" = 39.45
  dimension "d4" = 21.5
  dimension "d5" = 10.24
  constraint horizontal L0
  constraint vertical L1
  constraint horizontal L2
  constraint vertical L3
  constraint coincident L0.start L3.end
  constraint coincident L3 L4.start
  constraint perpendicular L3 L4
  constraint horizontal L5
  constraint vertical L6
  constraint horizontal L7
  constraint vertical L8
  constraint horizontal L9
  constraint vertical L10
  constraint horizontal L11
  constraint vertical L12
  constraint coincident L0 L10.end
  measures "d1" distance of L0.start L0.end
  measures "d2" distance of L0.start L2.end
  measures "d3" distance of L4.start L4.end
  measures "d4" distance of L5.start L7.end
  measures "d5" distance of L2.end L9.end
extrude "Extrude1" add sketch "Sketch1" along normal blind 4.8 makes body 1
extrude "Extrude2" add sketch "Sketch1" against normal blind 5.2 contours L1 L5 L6 L7 L8 bodies 1
extrude "Extrude3" add sketch "Sketch1" along normal blind 6.9 contours L0 L2 L3 L9 L10 L11 L12 bodies 1
chamfer "Chamfer1" distance 15 distance2 5 1 edges at (33.8, 14.85, 0) measured on face at (11.2667, 9.9, 0) on bodies 1
fillet "Fillet1" radius 3 1 edges at (39.45, 14.85, -5.2) on bodies 1
sketch "Sketch2" plane through (39.45, 0, 0) normal (1, 0, 0) x (0, 1, 0)
  line L0 (4.1, -2.2) -> (25.6, -2.2)
  line L1 (25.6, -2.2) -> (25.6, 4.8)
  line L2 (25.6, 4.8) -> (4.1, 4.8)
  line L3 (4.1, 4.8) -> (4.1, -2.2)
  circle A0 centre (24.3342, 3.2338) radius 0.9
  circle A1 centre (24.3342, 1.4338) radius 0.9
  line L4 (24.3342, 3.2338) -> (24.3342, 1.4338) construction
  circle A2 centre (12.4804, 3.5968) radius 0.9
  circle A3 centre (10.647, 3.5968) radius 0.9
  circle A4 centre (8.8137, 3.5968) radius 0.9
  circle A5 centre (6.9804, 3.5968) radius 0.9
  dimension "d17" = 1.8
  dimension "d18" = 1.8
  dimension "d19" = 1.8
  dimension "d20" = 1.8
  dimension "d23" = -5.5
  dimension "d24" = 0
  constraint coincident A0.centre L4.start
  constraint coincident A1.centre L4.end
  constraint parallel L1 L4
  measures "d17" diameter of A0
  measures "d18" diameter of A1
  measures "d19" distance of A0.centre A1.centre
  measures "d20" diameter of A2
extrude "Extrude4" add sketch "Sketch2" along normal blind 13 separate body contours A0 | A1 | A2 | A3 | A4 | A5 makes body 3 at (43.7833, 24.6374, 4.0812) makes body 3 at (48.1167, 24.6374, 0.5864) makes body 5 at (43.7833, 13.3759, 3.5072) makes body 2 at (43.7833, 11.5426, 3.5072) makes body 4 at (43.7833, 9.7092, 3.5072) makes body 6 at (43.7833, 7.8759, 3.5072)
sketch "Sketch3" plane through (0, 0, 0) normal (-1, 0, 0) x (0, -1, 0)
  line L0 (-25.6, 0) -> (0, 0)
  line L1 (0, 0) -> (0, 6.9)
  line L2 (0, 6.9) -> (-25.6, 6.9)
  line L3 (-25.6, 6.9) -> (-25.6, 0)
  circle A0 centre (-1.9297, 1.5518) radius 0.9
  circle A1 centre (-7.4297, 1.5518) radius 0.9
  circle A2 centre (-12.9297, 1.5518) radius 0.9
  circle A3 centre (-18.4297, 1.5518) radius 0.9
  circle A4 centre (-23.9297, 1.5518) radius 0.9
  dimension "d27" = 1.8
  dimension "d30" = -22
  dimension "d31" = 0
  measures "d27" diameter of A0
extrude "Extrude5" add sketch "Sketch3" along normal blind 15 contours A0 | A1 | A3 | A4 bodies 1
equation "d8 = -10 mm + 4.8 mm"
equation "d18 = d17"

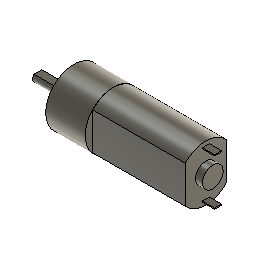
design "16mm diameter 1000rpm 12v motor"
Autodesk Fusion 360 part; units mm, degrees
sketch "Sketch1" plane through (0, 0, 0) normal (1, 0, 0) x (0, 1, 0)
  line L0 (-5.875, 5.3188) -> (-5.875, -5.3188)
  line L1 (5.875, -5.3188) -> (5.875, 5.3188)
  arc A0 (5.875, 5.3188) -> (-5.875, 5.3188) centre (0, 0) ccw
  arc A1 (-5.875, -5.3188) -> (5.875, -5.3188) centre (0, 0) ccw
  dimension "d1" = 15.85
  constraint parallel L0 L1
  constraint coincident L0.end A0
  constraint concentric A0 A1
  measures "d1" diameter of A0
extrude "Extrude1" add sketch "Sketch1" along normal blind 26.45
sketch "Sketch2" plane through (0, 0, 0) normal (-1, 0, 0) x (0, -1, 0)
  arc A0 (-5.875, -5.3188) -> (5.875, -5.3188) centre (0, 0) ccw
  line L0 (5.875, -5.3188) -> (5.875, 5.3188)
  arc A1 (5.875, 5.3188) -> (-5.875, 5.3188) centre (0, 0) ccw
  line L1 (-5.875, 5.3188) -> (-5.875, -5.3188)
  circle A2 centre (0, 0) radius 8
  dimension "d5" = 16
  constraint concentric A0 A2
  measures "d5" diameter of A2
extrude "Extrude2" add sketch "Sketch2" along normal blind 11.29 contours A0 L0 A1 L1 | A2
sketch "Sketch3" plane through (-11.29, 0, 0) normal (-1, 0, 0) x (0, -1, 0)
  circle A0 centre (0, 0) radius 8
  circle A1 centre (0, 0) radius 3
  dimension "d8" = 6
  constraint concentric A0 A1
  measures "d8" diameter of A1
extrude "Extrude3" add sketch "Sketch3" along normal blind 2.57 contours A1
sketch "Sketch4" plane through (-13.86, 0, 0) normal (-1, 0, 0) x (0, -1, 0)
  circle A0 centre (0, 0) radius 3
  circle A1 centre (0, 0) radius 1.5
  line L0 (0, -1.5) -> (0, 1) construction
  line L1 (1.118, 1) -> (-1.118, 1)
  dimension "d11" = 3
  dimension "d12" = 2.5
  constraint concentric A0 A1
  constraint coincident A1 L0.start
  constraint vertical L0
  constraint coincident A1 L1.start
  constraint coincident A1 L1.end
  constraint perpendicular L0 L1
  measures "d11" diameter of A1
  measures "d12" distance of L0.start L0.end
extrude "Extrude4" add sketch "Sketch4" along normal blind 7.68 contours A1 L1 picked at (-0.1071, 0.1783)
sketch "Sketch5" plane through (26.45, 0, 0) normal (1, 0, 0) x (0, 1, 0)
  arc A0 (-5.875, -5.3188) -> (5.875, -5.3188) centre (0, 0) ccw
  line L0 (5.875, -5.3188) -> (5.875, 5.3188)
  arc A1 (5.875, 5.3188) -> (-5.875, 5.3188) centre (0, 0) ccw
  line L1 (-5.875, 5.3188) -> (-5.875, -5.3188)
  circle A2 centre (0, 0) radius 2.95
  line L2 (0, 0) -> (0, 6.75) construction
  line L3 (1, 6.45) -> (-1, 6.45)
  line L4 (-1, 6.45) -> (-1, 6.75)
  line L5 (1, 6.75) -> (1, 6.45)
  line L6 (1, 6.45) -> (0, 6.75) construction
  line L7 (-1, 6.45) -> (0, 6.75) construction
  line L8 (-1, 6.75) -> (1, 6.75)
  line L9 (0, 0) -> (0.6035, 0) construction
  line L10 (-1, -6.45) -> (0, -6.75) construction
  line L11 (-1, -6.45) -> (-1, -6.75)
  line L12 (1, -6.45) -> (0, -6.75) construction
  line L13 (1, -6.75) -> (1, -6.45)
  line L14 (1, -6.45) -> (-1, -6.45)
  line L15 (-1, -6.75) -> (1, -6.75)
  point P0 (0, 6.75)
  point P1 (0, -6.75)
  dimension "d15" = 5.9
  dimension "d16" = 6.75
  constraint coincident A0.centre A1.centre
  constraint vertical L2
  constraint horizontal L3
  constraint perpendicular L3 L4
  constraint parallel L4 L5
  constraint coincident L6 P0
  constraint coincident L7 P0
  constraint coincident P0 L2.end
  constraint perpendicular L2 L9
  constraint symmetric P0 L9 P1
  constraint symmetric L3.start L9 L12.start
  constraint symmetric L3.end L9 L10.start
  constraint symmetric L4.end L9 L11.end
  constraint symmetric L5.start L9 L13.start
  measures "d15" diameter of A2
  measures "d16" distance of A0.centre P0
extrude "Extrude5" add sketch "Sketch5" along normal blind 2 contours A2 | L3 L4 L5 L8 | L11 L13 L14 L15
extrude "Extrude6" add 2 faces at (28.45, 0.3333, 6.55) (28.45, 0.3333, -6.65) along direction (1, 0, 0) blind 1.5
equation "d16 = ( 13.5 / 2 ) * 1 mm"

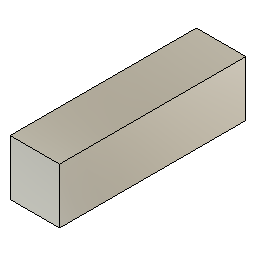
design "500mah battery"
Autodesk Fusion 360 part; units mm, degrees
sketch "Sketch1" plane through (0, 0, 0) normal (0, 0, 1) x (1, 0, 0)
  line L0 (0, 0) -> (17, 0)
  line L1 (17, 0) -> (17, 64)
  line L2 (17, 64) -> (0, 64)
  line L3 (0, 64) -> (0, 0)
  dimension "d1" = 17
  dimension "d2" = 64
  constraint horizontal L0
  constraint vertical L1
  constraint horizontal L2
  constraint vertical L3
  constraint coincident L0.start L3.end
  measures "d1" distance of L0.start L0.end
  measures "d2" distance of L0.start L2.end
extrude "Extrude1" add sketch "Sketch1" along normal blind 19
